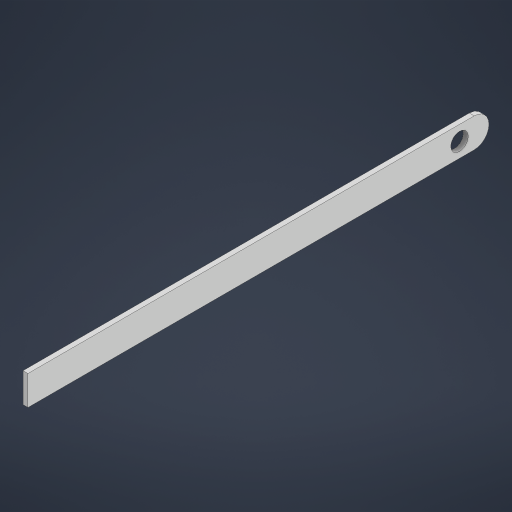
# Autodesk Inventor part: Arm
Saved by Autodesk Inventor 2023 (Build 270158000, 158)
## iProperties
Created: 2023-01-21
Part Number: Arm
Material: Generic
Document SubType Name: Modeling
Designer: Terrence
Density: 1 g/cm^3
Appearance: Default
Author: Terrence
Autodesk Inventor part; units mm, degrees
ref_plane "YZ Plane" through (0, 0, 0) normal (1, 0, 0) x (0, 1, 0)
ref_plane "XZ Plane" through (0, 0, 0) normal (0, 1, 0) x (-1, 0, 0)
ref_plane "XY Plane" through (0, 0, 0) normal (0, 0, 1) x (1, 0, 0)
sketch "Sketch1" plane through (0, 0, 0) normal (1, 0, 0) x (0, 1, 0)
  line L0 (0, 0) -> (76.2, 0)
  line L1 (76.2, 0) -> (76.2, -1193.8)
  line L2 (76.2, -1193.8) -> (0, -1193.8)
  line L3 (0, -1193.8) -> (0, 0)
  dimension "d0" = 76.2
  dimension "d1" = 1193.8
  constraints: 8 end point, 2 parallel, 1 horizontal, 1 perpendicular
  measures "d0" distance of L1.end L2.end
  measures "d1" distance of L0.end L1.end
extrude "Extrusion1" add sketch "Sketch1" along normal blind 12.7
sketch "Sketch2" plane through (12.7, 0, 0) normal (1, 0, 0) x (0, 0, -1)
  line L0 (1193.8, 76.2) -> (0, 76.2) projected
  line L1 (1117.6, 76.2) -> (1117.6, 0) construction
  line L2 (0, 0) -> (1193.8, 0) projected
  circle A0 centre (1117.6, 38.1) radius 22.5482
  dimension "d5" = 1117.6
  constraints: 2 end point, 2 point on line, 1 centre point, 1 midpoint, 1 perpendicular
  measures "d5" distance from line of L2.start L1
extrude "Extrusion2" cut sketch "Sketch2" against normal through all
fillet "Fillet1" radius 38.1 2 edges at (6.35, 76.2, -1193.8) (6.35, 0, -1193.8)
body "Solid1"
